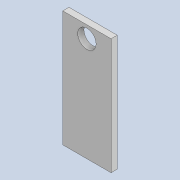
# Autodesk Inventor part: Base_cortadora
Saved by Autodesk Inventor 2021 (Build 250183000, 183)
## iProperties
Created: 2021-04-30
Part Number: Base_cortadora
Material: Genérico
Document SubType Name: Modeling
Designer: Admin
Density: 1 g/cm^3
Appearance: Valor por defecto
Author: Admin
Autodesk Inventor part; units mm, degrees
ref_plane "YZ Plane" through (0, 0, 0) normal (1, 0, 0) x (0, 1, 0)
ref_plane "XZ Plane" through (0, 0, 0) normal (0, 1, 0) x (-1, 0, 0)
ref_plane "XY Plane" through (0, 0, 0) normal (0, 0, 1) x (1, 0, 0)
sketch "Boceto1" plane through (0, 0, 0) normal (0, 0, 1) x (1, 0, 0)
  line L0 (0, 0) -> (50, 0)
  line L1 (50, 0) -> (50, 120)
  line L2 (50, 120) -> (0, 120)
  line L3 (0, 120) -> (0, 0)
  dimension "d0" = 50
  dimension "d1" = 120
  constraints: 8 end point, 2 parallel, 1 horizontal, 1 perpendicular
  measures "d0" distance of L2.end L1.end
  measures "d1" distance of L1.end L0.end
extrude "Extrusión1" add sketch "Boceto1" along normal blind 6.4
sketch "Boceto2" plane through (0, 0, 6.4) normal (0, 0, 1) x (1, 0, 0)
  line L0 (50, 120) -> (0, 120) projected
  line L1 (25, 120) -> (25, 117)
  line L2 (25, 117) -> (25, 107.5)
  circle A0 centre (25, 107.5) radius 9.5
  point P0 (0, 0)
  dimension "d4" = 3
  dimension "d5" = 9.5
  dimension "d6" = 19
  constraints: 4 end point, 1 centre point, 1 coincident, 1 midpoint, 1 point on line, 1 vertical
  measures "d4" distance of L1.start L1.end
  measures "d5" distance of L1.end L2.end
  measures "d6" diameter of A0
extrude "Extrusión2" cut sketch "Boceto2" against normal through all
